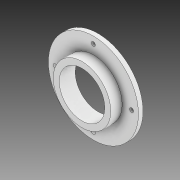
# Autodesk Inventor part: 2209B_Tube Flange Inner_V1
Saved by Autodesk Inventor 2020 (Build 240168000, 168)
## iProperties
Created: 2019-10-22
Part Number: 2209B_Tube Flange Inner_V1
Material: ABS Plastic
Document SubType Name: Modeling
Designer: RFLab
Density: 1.06 g/cm^3
Appearance: Smooth - White
Author: RFLab
Autodesk Inventor part; units mm, degrees
ref_plane "YZ Plane" through (0, 0, 0) normal (1, 0, 0) x (0, 1, 0)
ref_plane "XZ Plane" through (0, 0, 0) normal (0, 1, 0) x (-1, 0, 0)
ref_plane "XY Plane" through (0, 0, 0) normal (0, 0, 1) x (1, 0, 0)
sketch "Sketch1" plane through (0, 0, 0) normal (0, 0, 1) x (1, 0, 0)
  circle A0 centre (0, 0) radius 25.2
  dimension "d0" = 50.4
  constraints: 1 centre point, 1 coincident
  measures "d0" diameter of A0
extrude "Extrusion1" add sketch "Sketch1" along normal blind 10
sketch "Sketch2" plane through (0, 0, 10) normal (0, 0, 1) x (1, 0, 0)
  circle A0 centre (0, 0) radius 25.2 projected
  circle A1 centre (0, 0) radius 7
  dimension "d3" = 14
  constraints: 1 centre point, 1 coincident
  measures "d3" diameter of A1
extrude "Extrusion2" add sketch "Sketch2" along normal blind 6 contours A1
sketch "Sketch3" plane through (0, 0, 0) normal (0, 0, -1) x (-1, 0, 0)
  circle A0 centre (0, 0) radius 7 projected
  circle A1 centre (0, 0) radius 39.5
  dimension "d6" = 79
  constraints: 1 centre point, 1 coincident
  measures "d6" diameter of A1
extrude "Extrusion3" add sketch "Sketch3" along normal blind 4 contours A0 | A1
sketch "Sketch4" plane through (0, 0, 16) normal (0, 0, 1) x (1, 0, 0)
  circle A0 centre (0, 0) radius 7 projected
  circle A1 centre (0, 0) radius 4
  dimension "d9" = 8
  constraints: 1 centre point, 1 coincident
  measures "d9" diameter of A1
extrude "Extrusion4" cut sketch "Sketch4" against normal through all contours A1
sketch "Sketch5" plane through (0, 0, 0) normal (0, 0, 1) x (1, 0, 0)
  circle A0 centre (0, 0) radius 4 projected
  line L0 (0, 0) -> (0, 39.5)
  circle A1 centre (0, 0) radius 39.5 projected
  line L1 (0, 0) -> (0, -39.5)
  circle A2 centre (0, 0) radius 39.5 projected
  circle A3 centre (0, 0) radius 4 projected
  line L2 (0, 0) -> (38.7035, 0)
  circle A4 centre (0, 0) radius 7 projected
  line L3 (0, 0) -> (-39.5, 0)
  circle A5 centre (0, 0) radius 7 projected
  circle A6 centre (0, -33.5) radius 1.75
  circle A7 centre (33.5, 0) radius 1.75
  circle A8 centre (0, 33.5) radius 1.75
  circle A9 centre (-33.5, 0) radius 1.75
  circle A10 centre (0, 0) radius 33.5
  dimension "d13" = 3.5
  dimension "d19" = 67
  constraints: 8 end point, 6 point on circle, 5 centre point, 5 point on line, 3 equal radius, 2 horizontal, 1 coincident, 1 vertical, 1 vertical alignment, 1 other
  measures "d13" diameter of A6
  measures "d19" diameter of A10
extrude "Extrusion5" cut sketch "Sketch5" against normal through all contours A7 A10 L2 | L2 A10 A7 | A8 A10 L0 | L0 A10 A8 | A6 A10 L1 | L1 A10 A6 | A10 A7 L2 | L2 A7 A10 | A9 A10 L3 | L3 A10 A9 | A10 A8 L0 | L0 A8 A10 | A10 A6 L1 | L1 A6 A10 | A10 A9 L3 | L3 A9 A10
sketch "Sketch7" plane through (0, 0, -4) normal (0, 0, -1) x (-1, 0, 0)
  circle A0 centre (0, 0) radius 20
  dimension "d20" = 40
  constraints: 1 centre point, 1 coincident
  measures "d20" diameter of A0
extrude "Extrusion7" cut sketch "Sketch7" against normal blind 75
body "Solid1"
